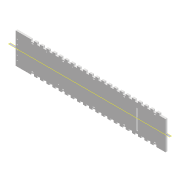
# Autodesk Inventor part: 10_Baseplate_Simmo_side1
Saved by Autodesk Inventor 2022.5 (Build 265521000, 521)
## iProperties
Created: 2022-08-04
Part Number: 10_Baseplate_Simmo_side1
Material: Generic
Document SubType Name: Modeling
Designer: wanghaoran
Density: 1 g/cm^3
Appearance: Default
Author: wanghaoran
Autodesk Inventor part; units mm, degrees
ref_plane "YZ Plane" through (0, 0, 0) normal (1, 0, 0) x (0, 1, 0)
ref_plane "XZ Plane" through (0, 0, 0) normal (0, 1, 0) x (-1, 0, 0)
ref_plane "XY Plane" through (0, 0, 0) normal (0, 0, 1) x (1, 0, 0)
sketch "Sketch1" plane through (0, 0, 0) normal (0, 0, 1) x (1, 0, 0)
  line L0 (4.9654, 0) -> (4.9654, 6) projected
  line L1 (-450, -9) -> (-450, -67) projected
  line L2 (35.4762, 11) -> (35.4762, 17) projected
  line L3 (35.4762, 17) -> (-454.5238, 17)
  line L4 (-454.5238, 17) -> (-454.5238, -83)
  line L5 (-454.5238, -83) -> (35.4762, -83)
  line L6 (35.4762, -83) -> (35.4762, 17)
  point P0 (-450, -9)
  point P1 (-450, -67)
  dimension "d26" = 490
  dimension "d27" = 100
  constraints: 8 end point, 2 parallel, 1 horizontal, 1 perpendicular
  measures "d26" distance of L5.end L4.end
  measures "d27" distance of L4.end L3.end
extrude "Extrusion1" add sketch "Sketch1" along normal blind 6
sketch "Sketch2" plane through (0, 0, 6) normal (0, 0, 1) x (1, 0, 0)
  line L0 (-14.5238, 11) -> (-14.5238, 17) projected
  line L1 (-24.5238, 17) -> (-14.5238, 17) projected
  line L2 (-24.5238, 17) -> (-24.5238, 11) projected
  line L3 (-24.5238, 11) -> (-14.5238, 11) projected
  line L4 (-14.5238, 17) -> (-14.4238, 17)
  line L5 (-14.4238, 17) -> (-14.4238, 11)
  line L6 (-14.4238, 11) -> (-14.5238, 11)
  line L7 (-14.5238, 11) -> (-14.5238, 17)
  line L8 (-24.5238, 17) -> (-24.6238, 17)
  line L9 (-24.6238, 17) -> (-24.6238, 11)
  line L10 (-24.6238, 11) -> (-24.5238, 11)
  line L11 (-24.5238, 11) -> (-24.5238, 17)
  point P0 (0, 0)
  point P1 (-14.5238, 11)
  dimension "d5" = 0.1
  dimension "d6" = 0.1
  constraints: 16 end point, 4 parallel, 2 horizontal, 2 perpendicular, 1 point on line
  measures "d5" distance of L5.end L6.end
  measures "d6" distance of L10.end L9.end
extrude "Extrusion2" cut sketch "Sketch2" against normal blind 6
pattern_linear "Rectangular Pattern1" count 20 spacing 20 along (-1, 0, 0) of "Extrusion2"
ref_plane "Work Plane1" through (-454.5238, -33, 0) normal (0, -1, 0) x (1, 0, 0)
sketch "Sketch4" plane through (0, 0, 6) normal (0, 0, 1) x (1, 0, 0)
  circle A0 centre (-449.5238, -65.5) radius 1.6
  line L0 (-449.5238, -65.5) -> (-449.5238, -43)
  circle A1 centre (-449.5238, -50.5) radius 1.6
  circle A2 centre (-449.5238, -35.5) radius 1.6
  circle A3 centre (-449.5238, -20.5) radius 1.6
  circle A4 centre (-449.5238, -5.5) radius 1.6
  line L1 (-454.5238, -83) -> (35.4762, -83) projected
  line L2 (-454.5238, 17) -> (-454.5238, -83) projected
  point P0 (0, 0)
  dimension "d15" = 3.2
  dimension "d18" = 15
  dimension "d46" = 17.5
  dimension "d47" = 5
  constraints: 5 centre point, 2 end point, 1 vertical, 8 other
  measures "d15" diameter of A0
  measures "d18" distance of L0.start A1.centre
  measures "d46" distance from line of L1 L0.start
  measures "d47" distance from line of L2 L0.start
extrude "Extrusion4" cut sketch "Sketch4" against normal blind 6
pattern_linear "Rectangular Pattern3" count 2 spacing 20 along (1, 0, 0) of "Extrusion2"
sketch "Sketch5" plane through (0, 0, 6) normal (0, 0, 1) x (1, 0, 0)
  line L0 (15.4762, 11) -> (35.4762, 11) projected
  line L1 (15.4762, 17) -> (15.4762, 11) projected
  line L2 (15.4762, 17) -> (35.4762, 17) projected
  line L3 (35.4762, 11) -> (35.4762, 17) projected
  point P0 (0, 0)
extrude "Extrusion5" cut sketch "Sketch5" against normal through all
mirror "Mirror3" about plane through (-454.5238, -33, 0) normal (0, -1, 0) of "Extrusion2", "Rectangular Pattern1"
mirror "Mirror4" about plane through (-454.5238, -33, 0) normal (0, -1, 0) of "Extrusion2", "Rectangular Pattern3"
sketch "Sketch6" plane through (0, 0, 6) normal (0, 0, 1) x (1, 0, 0)
  line L0 (3.2262, 5.6) -> (-2.2738, 5.6)
  line L1 (-2.2738, 5.6) -> (-2.2738, 8)
  line L2 (-2.2738, 8) -> (3.2262, 8)
  line L3 (3.2262, 8) -> (3.2262, 5.6)
  line L4 (-4.6238, 11) -> (-4.6238, 17) projected
  line L5 (5.5762, 11) -> (-4.6238, 11) projected
  line L6 (-102.2738, 8) -> (-96.7738, 8)
  line L7 (-96.7738, 5.6) -> (-102.2738, 5.6)
  line L8 (-102.2738, 5.6) -> (-102.2738, 8)
  line L9 (-96.7738, 8) -> (-96.7738, 5.6)
  line L10 (-202.2738, 8) -> (-196.7738, 8)
  line L11 (-196.7738, 5.6) -> (-202.2738, 5.6)
  line L12 (-202.2738, 5.6) -> (-202.2738, 8)
  line L13 (-196.7738, 8) -> (-196.7738, 5.6)
  line L14 (-302.2738, 8) -> (-296.7738, 8)
  line L15 (-296.7738, 5.6) -> (-302.2738, 5.6)
  line L16 (-302.2738, 5.6) -> (-302.2738, 8)
  line L17 (-296.7738, 8) -> (-296.7738, 5.6)
  line L18 (-402.2738, 8) -> (-396.7738, 8)
  line L19 (-396.7738, 5.6) -> (-402.2738, 5.6)
  line L20 (-402.2738, 5.6) -> (-402.2738, 8)
  line L21 (-396.7738, 8) -> (-396.7738, 5.6)
  point P0 (0, 0)
  dimension "d33" = 5.5
  dimension "d34" = 2.4
  dimension "d35" = 2.35
  dimension "d36" = 3
  dimension "d39" = 100
  constraints: 40 end point, 16 horizontal alignment, 10 parallel, 8 collinear, 1 horizontal, 1 perpendicular, 1 other
  measures "d33" distance of L1.end L2.end
  measures "d34" distance of L0.end L1.end
  measures "d35" distance between parallel lines of L4 L1
  measures "d39" distance of L1.end L6.start
extrude "Extrusion6" cut sketch "Sketch6" against normal through all
mirror "Mirror5" about plane through (-454.5238, -33, 0) normal (0, -1, 0) of "Extrusion6"
sketch "Sketch7" plane through (0, 0, 6) normal (0, 0, 1) x (1, 0, 0)
  line L0 (-49.606, -65.933) -> (-49.606, -17.933) projected
  line L1 (-51.5412, -65.933) -> (-49.606, -65.933) projected
  line L2 (-51.5412, -65.933) -> (-51.5412, -17.933) projected
  line L3 (-51.5412, -17.933) -> (-49.606, -17.933) projected
  line L4 (-55.5412, -4) -> (-59.5412, -4)
  line L5 (-59.5412, -4) -> (-59.5412, -69)
  line L6 (-59.5412, -69) -> (-55.5412, -69)
  line L7 (-55.5412, -69) -> (-55.5412, -4)
  line L8 (-54.4238, 11) -> (-64.6238, 11) projected
  point P0 (0, 0)
  point P1 (-46.2142, -12.933)
  dimension "d61" = 4
  dimension "d62" = 65
  dimension "d63" = 4
  dimension "d66" = 15
  constraints: 8 end point, 2 parallel, 1 horizontal, 1 perpendicular
  measures "d61" distance of L6.end L5.end
  measures "d62" distance of L5.end L4.end
  measures "d63" distance between parallel lines of L7 L2
  measures "d66" distance between parallel lines of L8 L4
extrude "Extrusion7" cut sketch "Sketch7" against normal through all contours L7 L6 L5 L4
sketch "Sketch8" plane through (0, 0, 6) normal (0, 0, 1) x (1, 0, 0)
  circle A0 centre (-268.0238, 6.5) radius 1.5 projected
  circle A1 centre (-353.7238, 6.5) radius 1.5 projected
  circle A2 centre (-315.1235, -66.1403) radius 1.55 projected
  point P0 (0, 0)
extrude "Extrusion8" cut sketch "Sketch8" against normal through all
body "Solid1"
